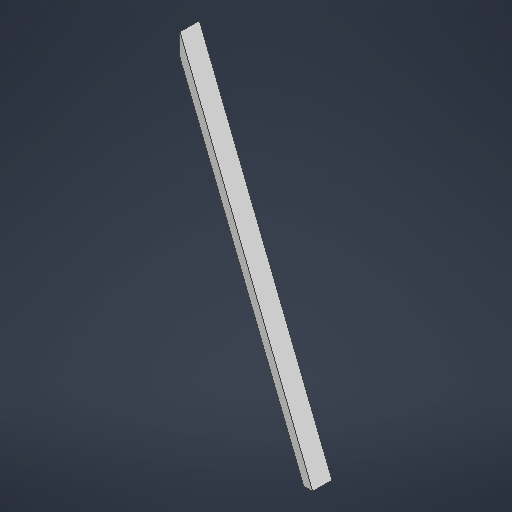
# Autodesk Inventor part: Part3
Saved by Autodesk Inventor 2026 (Build 300175000, 175)
## iProperties
Created: 2025-09-03
Part Number: Part3
Material: Generic
Document SubType Name: Modeling
Designer: trott
Density: 1 g/cm^3
Appearance: Default
Author: trott
Autodesk Inventor part; units mm, degrees
ref_plane "YZ Plane" through (0, 0, 0) normal (1, 0, 0) x (0, 1, 0)
ref_plane "XZ Plane" through (0, 0, 0) normal (0, 1, 0) x (-1, 0, 0)
ref_plane "XY Plane" through (0, 0, 0) normal (0, 0, 1) x (1, 0, 0)
sketch "Sketch1" plane through (0, 0, 0) normal (0, 0, 1) x (1, 0, 0)
  line L0 (0, 0) -> (0, 1524)
  line L1 (0, 0) -> (609.6, 0)
  line L2 (609.6, 0) -> (0, 1524)
  line L3 (609.6, 0) -> (574.225, -14.15)
  line L4 (0, 1524) -> (-35.375, 1509.85)
  line L5 (574.225, -14.15) -> (-35.375, 1509.85)
  point P0 (0, 1421.4126)
  point P1 (568.565, 0)
  dimension "d0" = 1524
  dimension "d1" = 609.6
  dimension "d2" = 38.1
  dimension "d3" = 38.1
  dimension "d4" = 90
  dimension "d5" = 90
  constraints: 12 end point, 1 horizontal, 1 vertical
  measures "d0" distance of L0.start L0.end
  measures "d1" distance of L0.start L1.end
  measures "d2" distance of L1.end L3.end
  measures "d3" distance of L0.end L4.end
  measures "d4" angle of L2 L4
  measures "d5" angle of L2 L3
extrude "Extrusion1" add sketch "Sketch1" along normal blind 88.9 contours L0 L2 L1 L5
body "Solid1"
